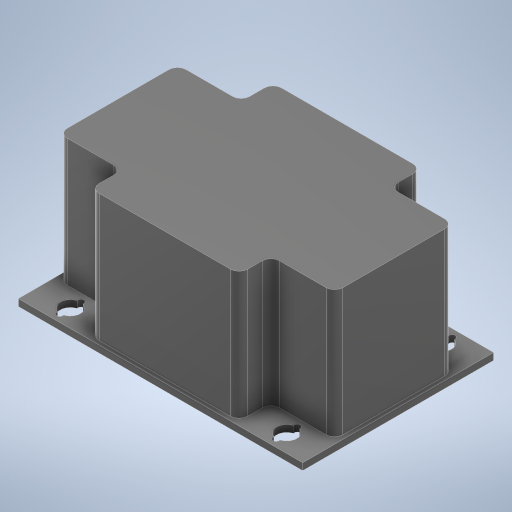
# Autodesk Inventor part: SUSTAINA-POWER-LOGGING-BOARD
Saved by Autodesk Inventor 2024.2 (Build 282272000, 272)
## iProperties
Created: 2024-01-24
Part Number: SUSTAINA-POWER-LOGGING-BOARD
Material: Acetal Resin, Black
Document SubType Name: Modeling
Designer: Masato Kubotera
Appearance: Smooth - Black
Surface Area: 123.153 cm^2
Volume: 52.2328 cm^3
Author: Masato Kubotera
Autodesk Inventor part; units mm, degrees
ref_plane "YZ Plane" through (0, 0, 0) normal (1, 0, 0) x (0, 1, 0)
ref_plane "XZ Plane" through (0, 0, 0) normal (0, 1, 0) x (-1, 0, 0)
ref_plane "XY Plane" through (0, 0, 0) normal (0, 0, 1) x (1, 0, 0)
sketch "Sketch1" plane through (0, 0, 0) normal (0, 0, 1) x (1, 0, 0)
  line L0 (22.5, 33.5) -> (-22.5, 33.5)
  line L1 (-22.5, 33.5) -> (-22.5, -33.5)
  line L2 (-22.5, -33.5) -> (22.5, -33.5)
  line L3 (22.5, -33.5) -> (22.5, 33.5)
  line L4 (22.5, 33.5) -> (-22.5, -33.5) construction
  line L5 (-22.5, 33.5) -> (22.5, -33.5) construction
  line L6 (-18.25, 25.5) -> (18.25, 25.5) construction
  line L7 (18.25, 25.5) -> (18.25, -25.5) construction
  line L8 (18.25, -25.5) -> (-18.25, -25.5) construction
  line L9 (-18.25, -25.5) -> (-18.25, 25.5) construction
  line L10 (-18.25, 25.5) -> (18.25, -25.5) construction
  line L11 (18.25, 25.5) -> (-18.25, -25.5) construction
  line L12 (22.5, 0) -> (-22.5, 0) construction
  line L13 (0, 33.5) -> (0, -33.5) construction
  circle A0 centre (18.25, 25.5) radius 2.4
  circle A1 centre (-18.25, 25.5) radius 2.4
  circle A2 centre (18.25, -25.5) radius 2.4
  circle A3 centre (-18.25, -25.5) radius 2.4
  line L14 (18.25, 32.5) -> (18.25, 18.5) construction
  line L15 (21.5, 17.5) -> (-21.5, 17.5)
  line L16 (-21.5, 17.5) -> (-21.5, -17.5)
  line L17 (-21.5, -17.5) -> (21.5, -17.5)
  line L18 (21.5, -17.5) -> (21.5, 17.5)
  line L19 (21.5, 17.5) -> (-21.5, -17.5) construction
  line L20 (-21.5, 17.5) -> (21.5, -17.5) construction
  line L21 (14, 17.5) -> (14, 32.5)
  line L22 (14, 32.5) -> (-14, 32.5)
  line L23 (-14, 32.5) -> (-14, 17.5)
  line L24 (14, -17.5) -> (14, -32.5)
  line L25 (14, -32.5) -> (-14, -32.5)
  line L26 (-14, -32.5) -> (-14, -17.5)
  arc A4 (15.9605, 26.2199) -> (15.9605, 24.7801) centre (15.75, 25.5) ccw
  arc A5 (20.5395, 24.7801) -> (20.5395, 26.2199) centre (20.75, 25.5) ccw
  arc A6 (15.9605, -24.7801) -> (15.9605, -26.2199) centre (15.75, -25.5) ccw
  arc A7 (20.5395, -26.2199) -> (20.5395, -24.7801) centre (20.75, -25.5) ccw
  arc A8 (-15.9605, 24.7801) -> (-15.9605, 26.2199) centre (-15.75, 25.5) ccw
  arc A9 (-20.5395, 26.2199) -> (-20.5395, 24.7801) centre (-20.75, 25.5) ccw
  arc A10 (-15.9605, -26.2199) -> (-15.9605, -24.7801) centre (-15.75, -25.5) ccw
  arc A11 (-20.5395, -24.7801) -> (-20.5395, -26.2199) centre (-20.75, -25.5) ccw
  point P0 (0, 0)
  point P1 (14, -17.5)
  point P2 (-14, -17.5)
  point P3 (21.5, 25.5)
  point P4 (15, 25.5)
  point P5 (20.5395, 26.2199)
  point P6 (20.5395, 24.7801)
  point P7 (20.5395, -24.7801)
  point P8 (20.5395, -26.2199)
  point P9 (15.9605, -26.2199)
  point P10 (15.9605, -24.7801)
  point P11 (-20.5395, -26.2199)
  point P12 (-20.5395, -24.7801)
  point P13 (-15.9605, -24.7801)
  point P14 (-15.9605, -26.2199)
  point P15 (-20.5395, 24.7801)
  point P16 (-20.5395, 26.2199)
  point P17 (-15.9605, 26.2199)
  point P18 (-15.9605, 24.7801)
  dimension "d0" = 45
  dimension "d1" = 67
  dimension "d19" = 4.8
  dimension "d33" = 51
  dimension "d34" = 36.5
  dimension "d38" = 1
  dimension "d43" = 1
  dimension "d44" = 1
  dimension "d46" = 6.5
  dimension "d47" = 1.5
  dimension "d48" = 1
  dimension "d50" = 16
  constraints: 54 end point, 28 symmetric about line, 20 point on circle, 12 centre point, 11 midpoint, 6 coincident, 6 parallel, 4 horizontal, 3 perpendicular, 3 point on line, 3 vertical, 13 other
  measures "d0" distance of L2.end L1.end
  measures "d1" distance of L1.end L0.end
  measures "d19" diameter of A0
  measures "d33" distance of L8.end L6.start
  measures "d34" distance of L7.end L8.end
  measures "d38" distance between parallel lines of L3 L18
  measures "d43" distance from line of L0 L14.start
  measures "d44" distance between parallel lines of L0 L22
  measures "d46" distance of point (21.5, 25.5) point (15, 25.5)
  measures "d47" diameter of A4
  measures "d48" distance from line of L3 point (21.5, 25.5)
  measures "d50" diameter of L0 L6
extrude "Extrusion1" add sketch "Sketch1" along normal blind 1.6 contours L3 L2 L1 L0 | L18 L17 L16 L15 | L15 L23 L22 L21 | L24 L25 L26 L17
extrude "Extrusion2" add sketch "Sketch1" along normal blind 31.6 contours L18 L17 L16 L15 | L15 L23 L22 L21 | L24 L25 L26 L17
fillet "Fillet1" radius 2 12 edges at (21.5, -17.5, 16.6) (21.5, 17.5, 16.6) (-21.5, -17.5, 16.6) (-21.5, 17.5, 16.6) (14, 17.5, 16.6) (14, -17.5, 16.6) (14, -32.5, 16.6) (-14, -32.5, 16.6) (-14, -17.5, 16.6) (-14, 17.5, 16.6) (-14, 32.5, 16.6) (14, 32.5, 16.6)
body "Solid1"
